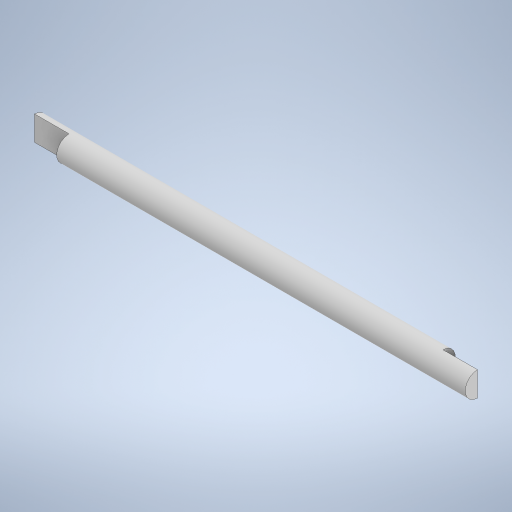
# Autodesk Inventor part: Aluminum_Rod_70mm
Saved by Autodesk Inventor 2023 (Build 270158030, 158C)
## iProperties
Created: 2022-06-17
Part Number: Aluminum_Rod_70mm
Material: Generic
Document SubType Name: Modeling
Designer: Mlees
Density: 1 g/cm^3
Appearance: Default
Author: Mlees
Autodesk Inventor part; units mm, degrees
ref_plane "YZ Plane" through (0, 0, 0) normal (1, 0, 0) x (0, 1, 0)
ref_plane "XZ Plane" through (0, 0, 0) normal (0, 1, 0) x (-1, 0, 0)
ref_plane "XY Plane" through (0, 0, 0) normal (0, 0, 1) x (1, 0, 0)
sketch "Sketch1" plane through (0, 0, 0) normal (1, 0, 0) x (0, 1, 0)
  circle A0 centre (0, 0) radius 2.5
  dimension "d0" = 5
  constraints: 1 centre point, 1 coincident
  measures "d0" diameter of A0
extrude "Extrusion1" add sketch "Sketch1" along normal blind 90
sketch "Sketch2" plane through (90, 0, 0) normal (1, 0, 0) x (0, 0, -1)
  circle A0 centre (0, 0) radius 2.5 projected
  arc A1 (0, -2.5) -> (0, 2.5) centre (0, 0) ccw
  line L0 (0, -2.5) -> (0, 2.5)
  constraints: 4 point on circle, 2 end point, 1 centre point, 1 vertical
extrude "Extrusion2" cut sketch "Sketch2" against normal blind 7 contours A0 L0 picked at (0.5196, 0.6515)
sketch "Sketch3" plane through (0, 0, 0) normal (-1, 0, 0) x (0, 0, 1)
  arc A0 (0, 2.5) -> (0, -2.5) centre (0, 0) ccw projected
  circle A1 centre (0, 0) radius 2.5 projected
  arc A2 (0, -2.5) -> (0, 2.5) centre (0, 0) ccw
  arc A3 (0, -2.5) -> (0, 2.5) centre (0, 0) ccw projected
  line L0 (0, -2.5) -> (0, 2.5)
  constraints: 3 point on circle, 2 end point, 1 centre point, 1 vertical
extrude "Extrusion3" cut sketch "Sketch3" against normal blind 7 contours A1 L0
body "Solid1"
